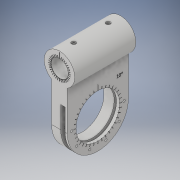
# Autodesk Inventor part: cam_holder_wrist_part
Saved by Autodesk Inventor 2019 (Build 230136000, 136)
## iProperties
Created: 2024-08-06
Part Number: cam_holder_wrist_part
Material: Generisch
Document SubType Name: Modeling
Designer: nic
Density: 1 g/cm^3
Appearance: Vorgabe
Author: nic
Autodesk Inventor part; units mm, degrees
ref_plane "YZ Plane" through (0, 0, 0) normal (1, 0, 0) x (0, 1, 0)
ref_plane "XY Plane" through (0, 0, 0) normal (0, 0, 1) x (1, 0, 0)
sketch "Skizze1" plane through (0, 0, 0) normal (1, 0, 0) x (0, 1, 0)
  line L0 (0, 0) -> (0, 35) construction
  circle A0 centre (0, 35) radius 35
  circle A1 centre (0, 35) radius 25.05
  dimension "d0" = 35
  dimension "d1" = 50.1
  constraints: 2 coincident, 2 end point, 1 centre point, 1 vertical, 1 vertical alignment, 2 other
  measures "d0" distance of L0.start L0.end
  measures "d1" diameter of A1
extrude "Extrusion1" add sketch "Skizze1" along normal blind 18
sketch "Skizze2" plane through (0, 0, 0) normal (0, 0, 1) x (1, 0, 0)
  line L0 (18, -35) -> (18, 35) construction
  line L1 (0, 35) -> (0, -35) construction
  line L2 (0, 35) -> (18, 35) projected
  line L3 (9, 35) -> (9, 60) construction
  circle A0 centre (9, 60) radius 10.05
  circle A1 centre (9, 60) radius 17.5
  point P0 (0, 0)
  dimension "d5" = 25
  dimension "d6" = 20.1
  dimension "d7" = 35
  constraints: 2 centre point, 2 coincident, 2 end point, 1 midpoint, 1 vertical
  measures "d5" distance of L3.start L3.end
  measures "d6" diameter of A0
  measures "d7" diameter of A1
extrude "Extrusion2" add sketch "Skizze2" along normal blind 70
sketch "Skizze3" plane through (0, 0, 0) normal (0, 0, 1) x (1, 0, 0)
  line L0 (18, -35) -> (18, 35) construction
  line L1 (0, 35) -> (0, -35) construction
  circle A0 centre (9, 60) radius 17.5 construction
  line L2 (18, -35) -> (18, 35) projected
  line L3 (18, 0) -> (0, 0)
  line L4 (0, 0) -> (0, 44.9917)
  line L5 (18, 44.9917) -> (18, 0)
  arc A1 (0, 44.9917) -> (18, 44.9917) centre (9, 60) ccw
  point P0 (0, 0)
  constraints: 6 end point, 2 point on circle, 1 centre point, 1 coincident, 1 horizontal, 1 midpoint, 1 parallel, 1 perpendicular, 2 other
extrude "Extrusion3" add sketch "Skizze3" along normal blind 70
sketch "Skizze4" plane through (0, 0, 0) normal (-1, 0, 0) x (0, 0, 1)
  line L0 (9.95, 0) -> (60.05, 0) projected
  circle A0 centre (35, 0) radius 25.05
  point P0 (0, 0)
  constraints: 1 centre point, 1 midpoint
extrude "Extrusion4" cut sketch "Skizze4" against normal through all
ref_plane "Arbeitsebene1" through (13, 0, 0) normal (1, 0, 0) x (0, 0, -1)
sketch "Skizze5" plane through (13, 0, 0) normal (1, 0, 0) x (0, 0, -1)
  circle A0 centre (-35, 0) radius 25.05 construction
  arc A1 (-70, 0) -> (0, 0) centre (-35, 0) ccw construction
  line L0 (0, 44.9917) -> (0, 0) construction
  line L1 (-70, 44.9917) -> (0, 44.9917) construction
  line L2 (-70, 0) -> (-70, 44.9917) construction
  circle A2 centre (-35, 0) radius 25.05
  arc A3 (-59.4438, 25.05) -> (-10.5562, 25.05) centre (-35, 0) ccw
  line L3 (-70, 0) -> (-70, 44.9917) projected
  line L4 (-70, 25.05) -> (0, 25.05)
  line L5 (0, 25.05) -> (0, 0)
  line L6 (-70, 0) -> (-70, 25.05)
  constraints: 6 end point, 4 point on circle, 3 point on line, 2 centre point, 2 coincident, 1 horizontal, 1 parallel, 1 perpendicular
extrude "Extrusion5" cut sketch "Skizze5" against normal blind 1.325 and the other way blind 1.325
sketch "Skizze6" plane through (13, 0, 0) normal (1, 0, 0) x (0, 0, -1)
  circle A0 centre (-35, 0) radius 25.05 construction
  arc A1 (-70, 0) -> (0, 0) centre (-35, 0) ccw construction
  line L0 (0, 44.9917) -> (0, 0) construction
  line L1 (-70, 44.9917) -> (0, 44.9917) construction
  line L2 (-70, 0) -> (-70, 44.9917) construction
  arc A2 (-70, 0) -> (0, 0) centre (-35, 0) ccw projected
  line L3 (-70, 25.05) -> (-70, 0) projected
  line L4 (0, 0) -> (0, 25.05) projected
  line L5 (-70, 25.05) -> (-35, 25.05) projected
  line L6 (-35, 25.05) -> (0, 25.05) projected
  line L7 (-65, 39.9917) -> (-5, 39.9917)
  line L8 (-5, 39.9917) -> (-5, 0)
  arc A3 (-65, 0) -> (-5, 0) centre (-35, 0) ccw
  line L9 (-65, 0) -> (-65, 39.9917)
  line L10 (-65, 25.05) -> (-5, 25.05)
  dimension "d19" = 5
  constraints: 8 end point, 4 point on line, 2 point on circle, 1 centre point, 1 vertical alignment, 3 other
  measures "d19" distance between parallel lines of L2 L9
extrude "Extrusion6" cut sketch "Skizze6" against normal blind 2.5 and the other way blind 2.5 contours L3 L5 L9 A3 L8 L6 L4 A2
ref_plane "Arbeitsebene2" through (0, 78, 0) normal (0, 1, 0) x (-1, 0, 0)
sketch "Skizze7" plane through (0, 78, 0) normal (0, 1, 0) x (-1, 0, 0)
  line L0 (-19.05, 70) -> (1.05, 70) projected
  line L1 (-9, 70) -> (-9, 0)
  point P0 (0, 0)
  point P1 (-9, 53.6501)
  point P2 (-9, 14.2598)
  constraints: 2 end point, 2 point on line, 1 midpoint, 1 vertical
hole "Bohrung1" at (9, 78, 53.6501) at (9, 78, 14.2598) direction (0, -1, 0) diameter 3.8 depth 10 tip angle 118 counterbore diameter 5 counterbore depth 2
sketch "Skizze8" plane through (0, 0, 70) normal (0, 0, 1) x (1, 0, 0)
  circle A0 centre (9, 60) radius 10.05 construction
  arc A1 (18, 44.9917) -> (0, 44.9917) centre (9, 60) ccw construction
  line L0 (8.75, 67.55) -> (9.25, 67.55)
  line L1 (9.25, 67.55) -> (9.25, 72.55)
  line L2 (9.25, 72.55) -> (8.75, 72.55)
  line L3 (8.75, 72.55) -> (8.75, 67.55)
  line L4 (8.75, 67.55) -> (9.25, 72.55) construction
  line L5 (9.25, 67.55) -> (8.75, 72.55) construction
  line L6 (7.4428, 67.3919) -> (7.9352, 67.4787)
  line L7 (7.9352, 67.4787) -> (7.0669, 72.4027)
  line L8 (7.0669, 72.4027) -> (6.5745, 72.3159)
  line L9 (6.5745, 72.3159) -> (7.4428, 67.3919)
  line L10 (7.4428, 67.3919) -> (7.0669, 72.4027) construction
  line L11 (7.9352, 67.4787) -> (6.5745, 72.3159) construction
  line L12 (6.1828, 67.0092) -> (6.6527, 67.1802)
  line L13 (6.6527, 67.1802) -> (4.9426, 71.8786)
  line L14 (4.9426, 71.8786) -> (4.4727, 71.7076)
  line L15 (4.4727, 71.7076) -> (6.1828, 67.0092)
  line L16 (6.1828, 67.0092) -> (4.9426, 71.8786) construction
  line L17 (6.6527, 67.1802) -> (4.4727, 71.7076) construction
  line L18 (5.0085, 66.4135) -> (5.4415, 66.6635)
  line L19 (5.4415, 66.6635) -> (2.9415, 70.9936)
  line L20 (2.9415, 70.9936) -> (2.5085, 70.7436)
  line L21 (2.5085, 70.7436) -> (5.0085, 66.4135)
  line L22 (5.0085, 66.4135) -> (2.9415, 70.9936) construction
  line L23 (5.4415, 66.6635) -> (2.5085, 70.7436) construction
  line L24 (3.9554, 65.6229) -> (4.3385, 65.9443)
  line L25 (4.3385, 65.9443) -> (1.1245, 69.7746)
  line L26 (1.1245, 69.7746) -> (0.7415, 69.4532)
  line L27 (0.7415, 69.4532) -> (3.9554, 65.6229)
  line L28 (3.9554, 65.6229) -> (1.1245, 69.7746) construction
  line L29 (4.3385, 65.9443) -> (0.7415, 69.4532) construction
  line L30 (3.0557, 64.6615) -> (3.3771, 65.0446)
  line L31 (3.3771, 65.0446) -> (-0.4532, 68.2585)
  line L32 (-0.4532, 68.2585) -> (-0.7746, 67.8755)
  line L33 (-0.7746, 67.8755) -> (3.0557, 64.6615)
  line L34 (3.0557, 64.6615) -> (-0.4532, 68.2585) construction
  line L35 (3.3771, 65.0446) -> (-0.7746, 67.8755) construction
  line L36 (2.3365, 63.5585) -> (2.5865, 63.9915)
  line L37 (2.5865, 63.9915) -> (-1.7436, 66.4915)
  line L38 (-1.7436, 66.4915) -> (-1.9936, 66.0585)
  line L39 (-1.9936, 66.0585) -> (2.3365, 63.5585)
  line L40 (2.3365, 63.5585) -> (-1.7436, 66.4915) construction
  line L41 (2.5865, 63.9915) -> (-1.9936, 66.0585) construction
  line L42 (1.8198, 62.3473) -> (1.9908, 62.8172)
  line L43 (1.9908, 62.8172) -> (-2.7076, 64.5273)
  line L44 (-2.7076, 64.5273) -> (-2.8786, 64.0574)
  line L45 (-2.8786, 64.0574) -> (1.8198, 62.3473)
  line L46 (1.8198, 62.3473) -> (-2.7076, 64.5273) construction
  line L47 (1.9908, 62.8172) -> (-2.8786, 64.0574) construction
  line L48 (1.5213, 61.0648) -> (1.6081, 61.5572)
  line L49 (1.6081, 61.5572) -> (-3.3159, 62.4255)
  line L50 (-3.3159, 62.4255) -> (-3.4027, 61.9331)
  line L51 (-3.4027, 61.9331) -> (1.5213, 61.0648)
  line L52 (1.5213, 61.0648) -> (-3.3159, 62.4255) construction
  line L53 (1.6081, 61.5572) -> (-3.4027, 61.9331) construction
  line L54 (1.45, 59.75) -> (1.45, 60.25)
  line L55 (1.45, 60.25) -> (-3.55, 60.25)
  line L56 (-3.55, 60.25) -> (-3.55, 59.75)
  line L57 (-3.55, 59.75) -> (1.45, 59.75)
  line L58 (1.45, 59.75) -> (-3.55, 60.25) construction
  line L59 (1.45, 60.25) -> (-3.55, 59.75) construction
  line L60 (1.6081, 58.4428) -> (1.5213, 58.9352)
  line L61 (1.5213, 58.9352) -> (-3.4027, 58.0669)
  line L62 (-3.4027, 58.0669) -> (-3.3159, 57.5745)
  line L63 (-3.3159, 57.5745) -> (1.6081, 58.4428)
  line L64 (1.6081, 58.4428) -> (-3.4027, 58.0669) construction
  line L65 (1.5213, 58.9352) -> (-3.3159, 57.5745) construction
  line L66 (1.9908, 57.1828) -> (1.8198, 57.6527)
  line L67 (1.8198, 57.6527) -> (-2.8786, 55.9426)
  line L68 (-2.8786, 55.9426) -> (-2.7076, 55.4727)
  line L69 (-2.7076, 55.4727) -> (1.9908, 57.1828)
  line L70 (1.9908, 57.1828) -> (-2.8786, 55.9426) construction
  line L71 (1.8198, 57.6527) -> (-2.7076, 55.4727) construction
  line L72 (2.5865, 56.0085) -> (2.3365, 56.4415)
  line L73 (2.3365, 56.4415) -> (-1.9936, 53.9415)
  line L74 (-1.9936, 53.9415) -> (-1.7436, 53.5085)
  line L75 (-1.7436, 53.5085) -> (2.5865, 56.0085)
  line L76 (2.5865, 56.0085) -> (-1.9936, 53.9415) construction
  line L77 (2.3365, 56.4415) -> (-1.7436, 53.5085) construction
  line L78 (3.3771, 54.9554) -> (3.0557, 55.3385)
  line L79 (3.0557, 55.3385) -> (-0.7746, 52.1245)
  line L80 (-0.7746, 52.1245) -> (-0.4532, 51.7415)
  line L81 (-0.4532, 51.7415) -> (3.3771, 54.9554)
  line L82 (3.3771, 54.9554) -> (-0.7746, 52.1245) construction
  line L83 (3.0557, 55.3385) -> (-0.4532, 51.7415) construction
  line L84 (4.3385, 54.0557) -> (3.9554, 54.3771)
  line L85 (3.9554, 54.3771) -> (0.7415, 50.5468)
  line L86 (0.7415, 50.5468) -> (1.1245, 50.2254)
  line L87 (1.1245, 50.2254) -> (4.3385, 54.0557)
  line L88 (4.3385, 54.0557) -> (0.7415, 50.5468) construction
  line L89 (3.9554, 54.3771) -> (1.1245, 50.2254) construction
  line L90 (5.4415, 53.3365) -> (5.0085, 53.5865)
  line L91 (5.0085, 53.5865) -> (2.5085, 49.2564)
  line L92 (2.5085, 49.2564) -> (2.9415, 49.0064)
  line L93 (2.9415, 49.0064) -> (5.4415, 53.3365)
  line L94 (5.4415, 53.3365) -> (2.5085, 49.2564) construction
  line L95 (5.0085, 53.5865) -> (2.9415, 49.0064) construction
  line L96 (6.6527, 52.8198) -> (6.1828, 52.9908)
  line L97 (6.1828, 52.9908) -> (4.4727, 48.2924)
  line L98 (4.4727, 48.2924) -> (4.9426, 48.1214)
  line L99 (4.9426, 48.1214) -> (6.6527, 52.8198)
  line L100 (6.6527, 52.8198) -> (4.4727, 48.2924) construction
  line L101 (6.1828, 52.9908) -> (4.9426, 48.1214) construction
  line L102 (7.9352, 52.5213) -> (7.4428, 52.6081)
  line L103 (7.4428, 52.6081) -> (6.5745, 47.6841)
  line L104 (6.5745, 47.6841) -> (7.0669, 47.5973)
  line L105 (7.0669, 47.5973) -> (7.9352, 52.5213)
  line L106 (7.9352, 52.5213) -> (6.5745, 47.6841) construction
  line L107 (7.4428, 52.6081) -> (7.0669, 47.5973) construction
  line L108 (9.25, 52.45) -> (8.75, 52.45)
  line L109 (8.75, 52.45) -> (8.75, 47.45)
  line L110 (8.75, 47.45) -> (9.25, 47.45)
  line L111 (9.25, 47.45) -> (9.25, 52.45)
  line L112 (9.25, 52.45) -> (8.75, 47.45) construction
  line L113 (8.75, 52.45) -> (9.25, 47.45) construction
  line L114 (10.5572, 52.6081) -> (10.0648, 52.5213)
  line L115 (10.0648, 52.5213) -> (10.9331, 47.5973)
  line L116 (10.9331, 47.5973) -> (11.4255, 47.6841)
  line L117 (11.4255, 47.6841) -> (10.5572, 52.6081)
  line L118 (10.5572, 52.6081) -> (10.9331, 47.5973) construction
  line L119 (10.0648, 52.5213) -> (11.4255, 47.6841) construction
  line L120 (11.8172, 52.9908) -> (11.3473, 52.8198)
  line L121 (11.3473, 52.8198) -> (13.0574, 48.1214)
  line L122 (13.0574, 48.1214) -> (13.5273, 48.2924)
  line L123 (13.5273, 48.2924) -> (11.8172, 52.9908)
  line L124 (11.8172, 52.9908) -> (13.0574, 48.1214) construction
  line L125 (11.3473, 52.8198) -> (13.5273, 48.2924) construction
  line L126 (12.9915, 53.5865) -> (12.5585, 53.3365)
  line L127 (12.5585, 53.3365) -> (15.0585, 49.0064)
  line L128 (15.0585, 49.0064) -> (15.4915, 49.2564)
  line L129 (15.4915, 49.2564) -> (12.9915, 53.5865)
  line L130 (12.9915, 53.5865) -> (15.0585, 49.0064) construction
  line L131 (12.5585, 53.3365) -> (15.4915, 49.2564) construction
  line L132 (14.0446, 54.3771) -> (13.6615, 54.0557)
  line L133 (13.6615, 54.0557) -> (16.8755, 50.2254)
  line L134 (16.8755, 50.2254) -> (17.2585, 50.5468)
  line L135 (17.2585, 50.5468) -> (14.0446, 54.3771)
  line L136 (14.0446, 54.3771) -> (16.8755, 50.2254) construction
  line L137 (13.6615, 54.0557) -> (17.2585, 50.5468) construction
  line L138 (14.9443, 55.3385) -> (14.6229, 54.9554)
  line L139 (14.6229, 54.9554) -> (18.4532, 51.7415)
  line L140 (18.4532, 51.7415) -> (18.7746, 52.1245)
  line L141 (18.7746, 52.1245) -> (14.9443, 55.3385)
  line L142 (14.9443, 55.3385) -> (18.4532, 51.7415) construction
  line L143 (14.6229, 54.9554) -> (18.7746, 52.1245) construction
  line L144 (15.6635, 56.4415) -> (15.4135, 56.0085)
  line L145 (15.4135, 56.0085) -> (19.7436, 53.5085)
  line L146 (19.7436, 53.5085) -> (19.9936, 53.9415)
  line L147 (19.9936, 53.9415) -> (15.6635, 56.4415)
  line L148 (15.6635, 56.4415) -> (19.7436, 53.5085) construction
  line L149 (15.4135, 56.0085) -> (19.9936, 53.9415) construction
  line L150 (16.1802, 57.6527) -> (16.0092, 57.1828)
  line L151 (16.0092, 57.1828) -> (20.7076, 55.4727)
  line L152 (20.7076, 55.4727) -> (20.8786, 55.9426)
  line L153 (20.8786, 55.9426) -> (16.1802, 57.6527)
  line L154 (16.1802, 57.6527) -> (20.7076, 55.4727) construction
  line L155 (16.0092, 57.1828) -> (20.8786, 55.9426) construction
  line L156 (16.4787, 58.9352) -> (16.3919, 58.4428)
  line L157 (16.3919, 58.4428) -> (21.3159, 57.5745)
  line L158 (21.3159, 57.5745) -> (21.4027, 58.0669)
  line L159 (21.4027, 58.0669) -> (16.4787, 58.9352)
  line L160 (16.4787, 58.9352) -> (21.3159, 57.5745) construction
  line L161 (16.3919, 58.4428) -> (21.4027, 58.0669) construction
  line L162 (16.55, 60.25) -> (16.55, 59.75)
  line L163 (16.55, 59.75) -> (21.55, 59.75)
  line L164 (21.55, 59.75) -> (21.55, 60.25)
  line L165 (21.55, 60.25) -> (16.55, 60.25)
  line L166 (16.55, 60.25) -> (21.55, 59.75) construction
  line L167 (16.55, 59.75) -> (21.55, 60.25) construction
  line L168 (16.3919, 61.5572) -> (16.4787, 61.0648)
  line L169 (16.4787, 61.0648) -> (21.4027, 61.9331)
  line L170 (21.4027, 61.9331) -> (21.3159, 62.4255)
  line L171 (21.3159, 62.4255) -> (16.3919, 61.5572)
  line L172 (16.3919, 61.5572) -> (21.4027, 61.9331) construction
  line L173 (16.4787, 61.0648) -> (21.3159, 62.4255) construction
  line L174 (16.0092, 62.8172) -> (16.1802, 62.3473)
  line L175 (16.1802, 62.3473) -> (20.8786, 64.0574)
  line L176 (20.8786, 64.0574) -> (20.7076, 64.5273)
  line L177 (20.7076, 64.5273) -> (16.0092, 62.8172)
  line L178 (16.0092, 62.8172) -> (20.8786, 64.0574) construction
  line L179 (16.1802, 62.3473) -> (20.7076, 64.5273) construction
  line L180 (15.4135, 63.9915) -> (15.6635, 63.5585)
  line L181 (15.6635, 63.5585) -> (19.9936, 66.0585)
  line L182 (19.9936, 66.0585) -> (19.7436, 66.4915)
  line L183 (19.7436, 66.4915) -> (15.4135, 63.9915)
  line L184 (15.4135, 63.9915) -> (19.9936, 66.0585) construction
  line L185 (15.6635, 63.5585) -> (19.7436, 66.4915) construction
  line L186 (14.6229, 65.0446) -> (14.9443, 64.6615)
  line L187 (14.9443, 64.6615) -> (18.7746, 67.8755)
  line L188 (18.7746, 67.8755) -> (18.4532, 68.2585)
  line L189 (18.4532, 68.2585) -> (14.6229, 65.0446)
  line L190 (14.6229, 65.0446) -> (18.7746, 67.8755) construction
  line L191 (14.9443, 64.6615) -> (18.4532, 68.2585) construction
  line L192 (13.6615, 65.9443) -> (14.0446, 65.6229)
  line L193 (14.0446, 65.6229) -> (17.2585, 69.4532)
  line L194 (17.2585, 69.4532) -> (16.8755, 69.7746)
  line L195 (16.8755, 69.7746) -> (13.6615, 65.9443)
  line L196 (13.6615, 65.9443) -> (17.2585, 69.4532) construction
  line L197 (14.0446, 65.6229) -> (16.8755, 69.7746) construction
  line L198 (12.5585, 66.6635) -> (12.9915, 66.4135)
  line L199 (12.9915, 66.4135) -> (15.4915, 70.7436)
  line L200 (15.4915, 70.7436) -> (15.0585, 70.9936)
  line L201 (15.0585, 70.9936) -> (12.5585, 66.6635)
  line L202 (12.5585, 66.6635) -> (15.4915, 70.7436) construction
  line L203 (12.9915, 66.4135) -> (15.0585, 70.9936) construction
  line L204 (11.3473, 67.1802) -> (11.8172, 67.0092)
  line L205 (11.8172, 67.0092) -> (13.5273, 71.7076)
  line L206 (13.5273, 71.7076) -> (13.0574, 71.8786)
  line L207 (13.0574, 71.8786) -> (11.3473, 67.1802)
  line L208 (11.3473, 67.1802) -> (13.5273, 71.7076) construction
  line L209 (11.8172, 67.0092) -> (13.0574, 71.8786) construction
  line L210 (10.0648, 67.4787) -> (10.5572, 67.3919)
  line L211 (10.5572, 67.3919) -> (11.4255, 72.3159)
  line L212 (11.4255, 72.3159) -> (10.9331, 72.4027)
  line L213 (10.9331, 72.4027) -> (10.0648, 67.4787)
  line L214 (10.0648, 67.4787) -> (11.4255, 72.3159) construction
  line L215 (10.5572, 67.3919) -> (10.9331, 72.4027) construction
  point P0 (0, 0)
  point P1 (9, 70.05)
  point P2 (7.2548, 69.8973)
  point P3 (5.5627, 69.4439)
  point P4 (3.975, 68.7036)
  point P5 (2.54, 67.6987)
  point P6 (1.3013, 66.46)
  point P7 (0.2964, 65.025)
  point P8 (-0.4439, 63.4373)
  point P9 (-0.8973, 61.7452)
  point P10 (-1.05, 60)
  point P11 (-0.8973, 58.2548)
  point P12 (-0.4439, 56.5627)
  point P13 (0.2964, 54.975)
  point P14 (1.3013, 53.54)
  point P15 (2.54, 52.3013)
  point P16 (3.975, 51.2964)
  point P17 (5.5627, 50.5561)
  point P18 (7.2548, 50.1027)
  point P19 (9, 49.95)
  point P20 (10.7452, 50.1027)
  point P21 (12.4373, 50.5561)
  point P22 (14.025, 51.2964)
  point P23 (15.46, 52.3013)
  point P24 (16.6987, 53.54)
  point P25 (17.7036, 54.975)
  point P26 (18.4439, 56.5627)
  point P27 (18.8973, 58.2548)
  point P28 (19.05, 60)
  point P29 (18.8973, 61.7452)
  point P30 (18.4439, 63.4373)
  point P31 (17.7036, 65.025)
  point P32 (16.6987, 66.46)
  point P33 (15.46, 67.6987)
  point P34 (14.025, 68.7036)
  point P35 (12.4373, 69.4439)
  point P36 (10.7452, 69.8973)
  dimension "d32" = 0.5
  dimension "d33" = 5
  dimension "d36" = 360
  constraints: 432 end point, 72 midpoint, 2 parallel, 1 horizontal, 1 perpendicular, 1 vertical alignment, 398 other
  measures "d32" distance of L2.end L1.end
  measures "d33" distance of L1.end L0.end
extrude "Extrusion7" cut sketch "Skizze8" against normal blind 0.5
sketch "Skizze9" plane through (0, 0, 70) normal (0, 0, 1) x (1, 0, 0)
  line L0 (9.25, 72.55) -> (9.25, 70.0469) projected
  line L1 (8.75, 70.0469) -> (8.75, 72.55) projected
  line L2 (8.75, 72.55) -> (9.25, 72.55) projected
  line L3 (11.5, 76) -> (6.5, 76) projected
  line L4 (8.75, 69.1) -> (9.25, 69.1)
  line L5 (9.25, 69.1) -> (9.25, 76)
  line L6 (9.25, 76) -> (8.75, 76)
  line L7 (8.75, 76) -> (8.75, 69.1)
  line L8 (8.75, 69.1) -> (9.25, 76) construction
  line L9 (9.25, 69.1) -> (8.75, 76) construction
  point P0 (0, 0)
  point P1 (9, 72.55)
  constraints: 12 end point, 3 midpoint, 2 parallel, 1 horizontal, 1 perpendicular, 1 point on line
extrude "Extrusion8" cut sketch "Skizze9" against normal blind 0.5
sketch "Skizze10" plane through (0, 0, 0) normal (0, 0, -1) x (-1, 0, 0)
  circle A0 centre (-9, 60) radius 10.05 projected
  circle A1 centre (-9, 60) radius 9.95
  point P0 (0, 0)
  dimension "d42" = 0.1
  constraints: 1 centre point
  measures "d42" radial gap between concentric circles of A0 A1
extrude "Extrusion9" add sketch "Skizze10" against normal up to surface (69.5 mm away)
sketch "Skizze11" plane through (18, 0, 0) normal (1, 0, 0) x (0, 0, -1)
  circle A0 centre (-35, 0) radius 25.05 projected
  line L0 (-35.25, 22.55) -> (-34.75, 22.55)
  line L1 (-34.75, 22.55) -> (-34.75, 27.55)
  line L2 (-34.75, 27.55) -> (-35.25, 27.55)
  line L3 (-35.25, 27.55) -> (-35.25, 22.55)
  line L4 (-65, 25.05) -> (-35, 25.05) projected
  line L5 (-35.25, 22.55) -> (-34.75, 27.55) construction
  line L6 (-34.75, 22.55) -> (-35.25, 27.55) construction
  line L7 (-39.162, 22.164) -> (-38.6696, 22.2508)
  line L8 (-38.6696, 22.2508) -> (-39.5378, 27.1749)
  line L9 (-39.5378, 27.1749) -> (-40.0302, 27.088)
  line L10 (-40.0302, 27.088) -> (-39.162, 22.164)
  line L11 (-39.162, 22.164) -> (-39.5378, 27.1749) construction
  line L12 (-38.6696, 22.2508) -> (-40.0302, 27.088) construction
  line L13 (-42.9475, 21.1046) -> (-42.4776, 21.2756)
  line L14 (-42.4776, 21.2756) -> (-44.1877, 25.974)
  line L15 (-44.1877, 25.974) -> (-44.6576, 25.803)
  line L16 (-44.6576, 25.803) -> (-42.9475, 21.1046)
  line L17 (-42.9475, 21.1046) -> (-44.1877, 25.974) construction
  line L18 (-42.4776, 21.2756) -> (-44.6576, 25.803) construction
  line L19 (-46.4915, 19.4039) -> (-46.0585, 19.6539)
  line L20 (-46.0585, 19.6539) -> (-48.5585, 23.984)
  line L21 (-48.5585, 23.984) -> (-48.9915, 23.734)
  line L22 (-48.9915, 23.734) -> (-46.4915, 19.4039)
  line L23 (-46.4915, 19.4039) -> (-48.5585, 23.984) construction
  line L24 (-46.0585, 19.6539) -> (-48.9915, 23.734) construction
  line L25 (-49.6864, 17.1136) -> (-49.3033, 17.435)
  line L26 (-49.3033, 17.435) -> (-52.5173, 21.2652)
  line L27 (-52.5173, 21.2652) -> (-52.9003, 20.9438)
  line L28 (-52.9003, 20.9438) -> (-49.6864, 17.1136)
  line L29 (-49.6864, 17.1136) -> (-52.5173, 21.2652) construction
  line L30 (-49.3033, 17.435) -> (-52.9003, 20.9438) construction
  line L31 (-52.435, 14.3033) -> (-52.1136, 14.6864)
  line L32 (-52.1136, 14.6864) -> (-55.9438, 17.9003)
  line L33 (-55.9438, 17.9003) -> (-56.2652, 17.5173)
  line L34 (-56.2652, 17.5173) -> (-52.435, 14.3033)
  line L35 (-52.435, 14.3033) -> (-55.9438, 17.9003) construction
  line L36 (-52.1136, 14.6864) -> (-56.2652, 17.5173) construction
  line L37 (-54.6539, 11.0585) -> (-54.4039, 11.4915)
  line L38 (-54.4039, 11.4915) -> (-58.734, 13.9915)
  line L39 (-58.734, 13.9915) -> (-58.984, 13.5585)
  line L40 (-58.984, 13.5585) -> (-54.6539, 11.0585)
  line L41 (-54.6539, 11.0585) -> (-58.734, 13.9915) construction
  line L42 (-54.4039, 11.4915) -> (-58.984, 13.5585) construction
  line L43 (-56.2756, 7.4776) -> (-56.1046, 7.9475)
  line L44 (-56.1046, 7.9475) -> (-60.803, 9.6576)
  line L45 (-60.803, 9.6576) -> (-60.974, 9.1877)
  line L46 (-60.974, 9.1877) -> (-56.2756, 7.4776)
  line L47 (-56.2756, 7.4776) -> (-60.803, 9.6576) construction
  line L48 (-56.1046, 7.9475) -> (-60.974, 9.1877) construction
  line L49 (-57.2508, 3.6696) -> (-57.164, 4.162)
  line L50 (-57.164, 4.162) -> (-62.088, 5.0302)
  line L51 (-62.088, 5.0302) -> (-62.1749, 4.5378)
  line L52 (-62.1749, 4.5378) -> (-57.2508, 3.6696)
  line L53 (-57.2508, 3.6696) -> (-62.088, 5.0302) construction
  line L54 (-57.164, 4.162) -> (-62.1749, 4.5378) construction
  line L55 (-57.55, -0.25) -> (-57.55, 0.25)
  line L56 (-57.55, 0.25) -> (-62.55, 0.25)
  line L57 (-62.55, 0.25) -> (-62.55, -0.25)
  line L58 (-62.55, -0.25) -> (-57.55, -0.25)
  line L59 (-57.55, -0.25) -> (-62.55, 0.25) construction
  line L60 (-57.55, 0.25) -> (-62.55, -0.25) construction
  line L61 (-57.164, -4.162) -> (-57.2508, -3.6696)
  line L62 (-57.2508, -3.6696) -> (-62.1749, -4.5378)
  line L63 (-62.1749, -4.5378) -> (-62.088, -5.0302)
  line L64 (-62.088, -5.0302) -> (-57.164, -4.162)
  line L65 (-57.164, -4.162) -> (-62.1749, -4.5378) construction
  line L66 (-57.2508, -3.6696) -> (-62.088, -5.0302) construction
  line L67 (-56.1046, -7.9475) -> (-56.2756, -7.4776)
  line L68 (-56.2756, -7.4776) -> (-60.974, -9.1877)
  line L69 (-60.974, -9.1877) -> (-60.803, -9.6576)
  line L70 (-60.803, -9.6576) -> (-56.1046, -7.9475)
  line L71 (-56.1046, -7.9475) -> (-60.974, -9.1877) construction
  line L72 (-56.2756, -7.4776) -> (-60.803, -9.6576) construction
  line L73 (-54.4039, -11.4915) -> (-54.6539, -11.0585)
  line L74 (-54.6539, -11.0585) -> (-58.984, -13.5585)
  line L75 (-58.984, -13.5585) -> (-58.734, -13.9915)
  line L76 (-58.734, -13.9915) -> (-54.4039, -11.4915)
  line L77 (-54.4039, -11.4915) -> (-58.984, -13.5585) construction
  line L78 (-54.6539, -11.0585) -> (-58.734, -13.9915) construction
  line L79 (-52.1136, -14.6864) -> (-52.435, -14.3033)
  line L80 (-52.435, -14.3033) -> (-56.2652, -17.5173)
  line L81 (-56.2652, -17.5173) -> (-55.9438, -17.9003)
  line L82 (-55.9438, -17.9003) -> (-52.1136, -14.6864)
  line L83 (-52.1136, -14.6864) -> (-56.2652, -17.5173) construction
  line L84 (-52.435, -14.3033) -> (-55.9438, -17.9003) construction
  line L85 (-49.3033, -17.435) -> (-49.6864, -17.1136)
  line L86 (-49.6864, -17.1136) -> (-52.9003, -20.9438)
  line L87 (-52.9003, -20.9438) -> (-52.5173, -21.2652)
  line L88 (-52.5173, -21.2652) -> (-49.3033, -17.435)
  line L89 (-49.3033, -17.435) -> (-52.9003, -20.9438) construction
  line L90 (-49.6864, -17.1136) -> (-52.5173, -21.2652) construction
  line L91 (-46.0585, -19.6539) -> (-46.4915, -19.4039)
  line L92 (-46.4915, -19.4039) -> (-48.9915, -23.734)
  line L93 (-48.9915, -23.734) -> (-48.5585, -23.984)
  line L94 (-48.5585, -23.984) -> (-46.0585, -19.6539)
  line L95 (-46.0585, -19.6539) -> (-48.9915, -23.734) construction
  line L96 (-46.4915, -19.4039) -> (-48.5585, -23.984) construction
  line L97 (-42.4776, -21.2756) -> (-42.9475, -21.1046)
  line L98 (-42.9475, -21.1046) -> (-44.6576, -25.803)
  line L99 (-44.6576, -25.803) -> (-44.1877, -25.974)
  line L100 (-44.1877, -25.974) -> (-42.4776, -21.2756)
  line L101 (-42.4776, -21.2756) -> (-44.6576, -25.803) construction
  line L102 (-42.9475, -21.1046) -> (-44.1877, -25.974) construction
  line L103 (-38.6696, -22.2508) -> (-39.162, -22.164)
  line L104 (-39.162, -22.164) -> (-40.0302, -27.088)
  line L105 (-40.0302, -27.088) -> (-39.5378, -27.1749)
  line L106 (-39.5378, -27.1749) -> (-38.6696, -22.2508)
  line L107 (-38.6696, -22.2508) -> (-40.0302, -27.088) construction
  line L108 (-39.162, -22.164) -> (-39.5378, -27.1749) construction
  line L109 (-34.75, -22.55) -> (-35.25, -22.55)
  line L110 (-35.25, -22.55) -> (-35.25, -27.55)
  line L111 (-35.25, -27.55) -> (-34.75, -27.55)
  line L112 (-34.75, -27.55) -> (-34.75, -22.55)
  line L113 (-34.75, -22.55) -> (-35.25, -27.55) construction
  line L114 (-35.25, -22.55) -> (-34.75, -27.55) construction
  line L115 (-30.838, -22.164) -> (-31.3304, -22.2508)
  line L116 (-31.3304, -22.2508) -> (-30.4622, -27.1749)
  line L117 (-30.4622, -27.1749) -> (-29.9698, -27.088)
  line L118 (-29.9698, -27.088) -> (-30.838, -22.164)
  line L119 (-30.838, -22.164) -> (-30.4622, -27.1749) construction
  line L120 (-31.3304, -22.2508) -> (-29.9698, -27.088) construction
  line L121 (-27.0525, -21.1046) -> (-27.5224, -21.2756)
  line L122 (-27.5224, -21.2756) -> (-25.8123, -25.974)
  line L123 (-25.8123, -25.974) -> (-25.3424, -25.803)
  line L124 (-25.3424, -25.803) -> (-27.0525, -21.1046)
  line L125 (-27.0525, -21.1046) -> (-25.8123, -25.974) construction
  line L126 (-27.5224, -21.2756) -> (-25.3424, -25.803) construction
  line L127 (-23.5085, -19.4039) -> (-23.9415, -19.6539)
  line L128 (-23.9415, -19.6539) -> (-21.4415, -23.984)
  line L129 (-21.4415, -23.984) -> (-21.0085, -23.734)
  line L130 (-21.0085, -23.734) -> (-23.5085, -19.4039)
  line L131 (-23.5085, -19.4039) -> (-21.4415, -23.984) construction
  line L132 (-23.9415, -19.6539) -> (-21.0085, -23.734) construction
  line L133 (-20.3136, -17.1136) -> (-20.6967, -17.435)
  line L134 (-20.6967, -17.435) -> (-17.4827, -21.2652)
  line L135 (-17.4827, -21.2652) -> (-17.0997, -20.9438)
  line L136 (-17.0997, -20.9438) -> (-20.3136, -17.1136)
  line L137 (-20.3136, -17.1136) -> (-17.4827, -21.2652) construction
  line L138 (-20.6967, -17.435) -> (-17.0997, -20.9438) construction
  line L139 (-17.565, -14.3033) -> (-17.8864, -14.6864)
  line L140 (-17.8864, -14.6864) -> (-14.0562, -17.9003)
  line L141 (-14.0562, -17.9003) -> (-13.7348, -17.5173)
  line L142 (-13.7348, -17.5173) -> (-17.565, -14.3033)
  line L143 (-17.565, -14.3033) -> (-14.0562, -17.9003) construction
  line L144 (-17.8864, -14.6864) -> (-13.7348, -17.5173) construction
  line L145 (-15.3461, -11.0585) -> (-15.5961, -11.4915)
  line L146 (-15.5961, -11.4915) -> (-11.266, -13.9915)
  line L147 (-11.266, -13.9915) -> (-11.016, -13.5585)
  line L148 (-11.016, -13.5585) -> (-15.3461, -11.0585)
  line L149 (-15.3461, -11.0585) -> (-11.266, -13.9915) construction
  line L150 (-15.5961, -11.4915) -> (-11.016, -13.5585) construction
  line L151 (-13.7244, -7.4776) -> (-13.8954, -7.9475)
  line L152 (-13.8954, -7.9475) -> (-9.197, -9.6576)
  line L153 (-9.197, -9.6576) -> (-9.026, -9.1877)
  line L154 (-9.026, -9.1877) -> (-13.7244, -7.4776)
  line L155 (-13.7244, -7.4776) -> (-9.197, -9.6576) construction
  line L156 (-13.8954, -7.9475) -> (-9.026, -9.1877) construction
  line L157 (-12.7492, -3.6696) -> (-12.836, -4.162)
  line L158 (-12.836, -4.162) -> (-7.912, -5.0302)
  line L159 (-7.912, -5.0302) -> (-7.8251, -4.5378)
  line L160 (-7.8251, -4.5378) -> (-12.7492, -3.6696)
  line L161 (-12.7492, -3.6696) -> (-7.912, -5.0302) construction
  line L162 (-12.836, -4.162) -> (-7.8251, -4.5378) construction
  line L163 (-12.45, 0.25) -> (-12.45, -0.25)
  line L164 (-12.45, -0.25) -> (-7.45, -0.25)
  line L165 (-7.45, -0.25) -> (-7.45, 0.25)
  line L166 (-7.45, 0.25) -> (-12.45, 0.25)
  line L167 (-12.45, 0.25) -> (-7.45, -0.25) construction
  line L168 (-12.45, -0.25) -> (-7.45, 0.25) construction
  line L169 (-12.836, 4.162) -> (-12.7492, 3.6696)
  line L170 (-12.7492, 3.6696) -> (-7.8251, 4.5378)
  line L171 (-7.8251, 4.5378) -> (-7.912, 5.0302)
  line L172 (-7.912, 5.0302) -> (-12.836, 4.162)
  line L173 (-12.836, 4.162) -> (-7.8251, 4.5378) construction
  line L174 (-12.7492, 3.6696) -> (-7.912, 5.0302) construction
  line L175 (-13.8954, 7.9475) -> (-13.7244, 7.4776)
  line L176 (-13.7244, 7.4776) -> (-9.026, 9.1877)
  line L177 (-9.026, 9.1877) -> (-9.197, 9.6576)
  line L178 (-9.197, 9.6576) -> (-13.8954, 7.9475)
  line L179 (-13.8954, 7.9475) -> (-9.026, 9.1877) construction
  line L180 (-13.7244, 7.4776) -> (-9.197, 9.6576) construction
  line L181 (-15.5961, 11.4915) -> (-15.3461, 11.0585)
  line L182 (-15.3461, 11.0585) -> (-11.016, 13.5585)
  line L183 (-11.016, 13.5585) -> (-11.266, 13.9915)
  line L184 (-11.266, 13.9915) -> (-15.5961, 11.4915)
  line L185 (-15.5961, 11.4915) -> (-11.016, 13.5585) construction
  line L186 (-15.3461, 11.0585) -> (-11.266, 13.9915) construction
  line L187 (-17.8864, 14.6864) -> (-17.565, 14.3033)
  line L188 (-17.565, 14.3033) -> (-13.7348, 17.5173)
  line L189 (-13.7348, 17.5173) -> (-14.0562, 17.9003)
  line L190 (-14.0562, 17.9003) -> (-17.8864, 14.6864)
  line L191 (-17.8864, 14.6864) -> (-13.7348, 17.5173) construction
  line L192 (-17.565, 14.3033) -> (-14.0562, 17.9003) construction
  line L193 (-20.6967, 17.435) -> (-20.3136, 17.1136)
  line L194 (-20.3136, 17.1136) -> (-17.0997, 20.9438)
  line L195 (-17.0997, 20.9438) -> (-17.4827, 21.2652)
  line L196 (-17.4827, 21.2652) -> (-20.6967, 17.435)
  line L197 (-20.6967, 17.435) -> (-17.0997, 20.9438) construction
  line L198 (-20.3136, 17.1136) -> (-17.4827, 21.2652) construction
  line L199 (-23.9415, 19.6539) -> (-23.5085, 19.4039)
  line L200 (-23.5085, 19.4039) -> (-21.0085, 23.734)
  line L201 (-21.0085, 23.734) -> (-21.4415, 23.984)
  line L202 (-21.4415, 23.984) -> (-23.9415, 19.6539)
  line L203 (-23.9415, 19.6539) -> (-21.0085, 23.734) construction
  line L204 (-23.5085, 19.4039) -> (-21.4415, 23.984) construction
  line L205 (-27.5224, 21.2756) -> (-27.0525, 21.1046)
  line L206 (-27.0525, 21.1046) -> (-25.3424, 25.803)
  line L207 (-25.3424, 25.803) -> (-25.8123, 25.974)
  line L208 (-25.8123, 25.974) -> (-27.5224, 21.2756)
  line L209 (-27.5224, 21.2756) -> (-25.3424, 25.803) construction
  line L210 (-27.0525, 21.1046) -> (-25.8123, 25.974) construction
  line L211 (-31.3304, 22.2508) -> (-30.838, 22.164)
  line L212 (-30.838, 22.164) -> (-29.9698, 27.088)
  line L213 (-29.9698, 27.088) -> (-30.4622, 27.1749)
  line L214 (-30.4622, 27.1749) -> (-31.3304, 22.2508)
  line L215 (-31.3304, 22.2508) -> (-29.9698, 27.088) construction
  line L216 (-30.838, 22.164) -> (-30.4622, 27.1749) construction
  line L217 (-34.75, 19.2227) -> (-35.25, 19.2227)
  line L218 (-35.25, 19.2227) -> (-35.25, 30.8773)
  line L219 (-35.25, 30.8773) -> (-34.75, 30.8773)
  line L220 (-34.75, 30.8773) -> (-34.75, 19.2227)
  line L221 (-34.75, 19.2227) -> (-35.25, 30.8773) construction
  line L222 (-35.25, 19.2227) -> (-34.75, 30.8773) construction
  point P0 (0, 0)
  dimension "d45" = 0.5
  dimension "d46" = 5
  dimension "d49" = 360
  constraints: 444 end point, 4 midpoint, 4 parallel, 2 horizontal, 2 perpendicular, 1 vertical alignment, 361 other
  measures "d45" distance of L2.end L1.end
  measures "d46" distance of L1.end L0.end
extrude "Extrusion10" cut sketch "Skizze11" against normal blind 0.5 contours A0 L164 L163 L166 | A0 L166 L165 L164 | L170 L169 L172 A0 | A0 L172 L171 L170 | L160 L159 L158 A0 | A0 L158 L157 L160 | L176 L175 L178 A0 | A0 L178 L177 L176 | L154 L153 L152 A0 | A0 L152 L151 L154 | L182 L181 L184 A0 | A0 L184 L183 L182 | L148 L147 L146 A0 | A0 L146 L145 L148 | L188 L187 L190 A0 | A0 L190 L189 L188 | L142 L141 L140 A0 | A0 L140 L139 L142 | L194 L193 L196 A0 | A0 L196 L195 L194 | L136 L135 L134 A0 | A0 L134 L133 L136 | L200 L199 L202 A0 | A0 L202 L201 L200 | L130 L129 L128 A0 | A0 L128 L127 L130 | L206 L205 L208 A0 | A0 L208 L207 L206 | L124 L123 L122 A0 | A0 L122 L121 L124 | L212 L211 L214 A0 | A0 L214 L213 L212 | L118 L117 L116 A0 | A0 L116 L115 L118 | L1 L0 L3 A0 | A0 L3 L2 L1 | L112 L111 L110 A0 | A0 L110 L109 L112 | L220 L217 L218 L0 | L2 L218 L219 L220 | L106 L105 L104 A0 | A0 L104 L103 L106 | L8 L7 L10 A0 | A0 L10 L4 L8 | L4 L10 L9 L8 | L100 L99 L98 A0 | A0 L98 L97 L100 | L14 L13 L16 A0 | A0 L16 L4 L14 | L4 L16 L15 L14 | L94 L93 L92 A0 | A0 L92 L91 L94 | L20 L19 L22 A0 | A0 L22 L21 L20 | L88 L87 L86 A0 | A0 L86 L85 L88 | L26 L25 L28 A0 | A0 L28 L27 L26 | L82 L81 L80 A0 | A0 L80 L79 L82 | L32 L31 L34 A0 | A0 L34 L33 L32 | L76 L75 L74 A0 | A0 L74 L73 L76 | L38 L37 L40 A0 | A0 L40 L39 L38 | L70 L69 L68 A0 | A0 L68 L67 L70 | L44 L43 L46 A0 | A0 L46 L45 L44 | L64 L63 L62 A0 | A0 L62 L61 L64 | L50 L49 L52 A0 | A0 L52 L51 L50 | L58 L57 L56 A0 | A0 L56 L55 L58
sketch "Skizze12" plane through (18, 0, 0) normal (1, 0, 0) x (0, 0, -1)
  line L0 (-13.6205, 29.8927) -> (-6.1014, 29.8927) construction
  line L1 (-6.1014, 29.8927) -> (-6.1014, 26.2481) construction
  line L2 (-6.1014, 26.2481) -> (-13.6205, 26.2481) construction
  line L3 (-13.6205, 26.2481) -> (-13.6205, 29.8927) construction
  line L4 (-11.3826, 26.3218) -> (-13.0901, 26.3218)
  line L5 (-13.0901, 26.3218) -> (-13.0901, 26.6792)
  line L6 (-13.0901, 26.6792) -> (-12.4548, 26.6792)
  line L7 (-12.4548, 26.6792) -> (-12.4548, 29.0248)
  line L8 (-12.4548, 29.0248) -> (-13.0901, 29.0248)
  line L9 (-13.0901, 29.0248) -> (-13.0901, 29.3453)
  spline S0 degree 2 poles (-13.0901, 29.3453) (-12.7299, 29.3453) (-12.3895, 29.5495) (-12.3668, 29.8332) knots 0 0 0 1 2 2 2
  line L10 (-12.3668, 29.8332) -> (-12.0038, 29.8332)
  line L11 (-12.0038, 29.8332) -> (-12.0038, 26.6792)
  line L12 (-12.0038, 26.6792) -> (-11.3826, 26.6792)
  line L13 (-11.3826, 26.6792) -> (-11.3826, 26.3218)
  spline S1 degree 2 poles (-8.5605, 28.0718) (-8.5605, 27.1302) (-9.1079, 26.2481) (-9.678, 26.2481) knots 0 0 0 1 2 2 2
  spline S2 degree 2 poles (-9.678, 26.2481) (-10.2566, 26.2481) (-10.7984, 27.1472) (-10.7984, 28.069) knots 0 0 0 1 2 2 2
  spline S3 degree 2 poles (-10.7984, 28.069) (-10.7984, 29.0163) (-10.2509, 29.8927) (-9.678, 29.8927) knots 0 0 0 1 2 2 2
  spline S4 degree 2 poles (-9.678, 29.8927) (-9.1022, 29.8927) (-8.5605, 28.9851) (-8.5605, 28.0718) knots 0 0 0 1 2 2 2
  spline S5 degree 2 poles (-9.1618, 27.0054) (-9.0937, 27.1784) (-9.037, 27.7116) (-9.037, 28.0718) knots 0 0 0 1 2 2 2
  spline S6 degree 2 poles (-9.037, 28.0718) (-9.037, 28.432) (-9.0937, 28.9624) (-9.1646, 29.1411) knots 0 0 0 1 2 2 2
  spline S7 degree 2 poles (-9.1646, 29.1411) (-9.2355, 29.3198) (-9.4823, 29.5041) (-9.678, 29.5041) knots 0 0 0 1 2 2 2
  spline S8 degree 2 poles (-9.678, 29.5041) (-9.8737, 29.5041) (-10.1261, 29.3198) (-10.1999, 29.1354) knots 0 0 0 1 2 2 2
  spline S9 degree 2 poles (-10.1999, 29.1354) (-10.2708, 28.9567) (-10.3219, 28.4122) (-10.3219, 28.069) knots 0 0 0 1 2 2 2
  spline S10 degree 2 poles (-10.3219, 28.069) (-10.3219, 27.7003) (-10.2765, 27.2067) (-10.2027, 27.0139) knots 0 0 0 1 2 2 2
  spline S11 degree 2 poles (-10.2027, 27.0139) (-10.1347, 26.8323) (-9.8822, 26.6366) (-9.678, 26.6366) knots 0 0 0 1 2 2 2
  spline S12 degree 2 poles (-9.678, 26.6366) (-9.4851, 26.6366) (-9.2327, 26.821) (-9.1618, 27.0054) knots 0 0 0 1 2 2 2
  spline S13 degree 2 poles (-6.3397, 28.9879) (-6.3397, 28.6107) (-6.8559, 28.0945) (-7.2331, 28.0945) knots 0 0 0 1 2 2 2
  spline S14 degree 2 poles (-7.2331, 28.0945) (-7.6075, 28.0945) (-8.1294, 28.6079) (-8.1294, 28.9879) knots 0 0 0 1 2 2 2
  spline S15 degree 2 poles (-8.1294, 28.9879) (-8.1294, 29.3652) (-7.6132, 29.8814) (-7.2331, 29.8814) knots 0 0 0 1 2 2 2
  spline S16 degree 2 poles (-7.2331, 29.8814) (-6.8559, 29.8814) (-6.3397, 29.3652) (-6.3397, 28.9879) knots 0 0 0 1 2 2 2
  spline S17 degree 2 poles (-6.7084, 28.9879) (-6.7084, 29.2148) (-7.009, 29.524) (-7.2331, 29.524) knots 0 0 0 1 2 2 2
  spline S18 degree 2 poles (-7.2331, 29.524) (-7.46, 29.524) (-7.7607, 29.2148) (-7.7607, 28.9879) knots 0 0 0 1 2 2 2
  spline S19 degree 2 poles (-7.7607, 28.9879) (-7.7607, 28.7582) (-7.4543, 28.4519) (-7.2331, 28.4519) knots 0 0 0 1 2 2 2
  spline S20 degree 2 poles (-7.2331, 28.4519) (-7.009, 28.4519) (-6.7084, 28.7639) (-6.7084, 28.9879) knots 0 0 0 1 2 2 2
  point P0 (0, 0)
  constraints: 2 other
extrude "Extrusion11" cut sketch "Skizze12" against normal blind 0.5
sketch "Skizze13" plane through (18, 0, 0) normal (1, 0, 0) x (0, 0, -1)
  line L0 (-11.3826, 26.6792) -> (-11.3826, 26.3218) construction
  line L1 (-11.3826, 26.3218) -> (-13.0901, 26.3218) construction
  line L2 (-13.0901, 26.3218) -> (-13.0901, 26.6792) construction
  line L3 (-13.0901, 26.6792) -> (-12.4548, 26.6792) construction
  line L4 (-12.4548, 26.6792) -> (-12.4548, 29.0248) construction
  line L5 (-12.4548, 29.0248) -> (-13.0901, 29.0248) construction
  line L6 (-13.0901, 29.0248) -> (-13.0901, 29.3453) construction
  line L7 (-12.3668, 29.8332) -> (-12.0038, 29.8332) construction
  line L8 (-12.0038, 29.8332) -> (-12.0038, 26.6792) construction
  line L9 (-12.0038, 26.6792) -> (-11.3826, 26.6792) construction
  line L10 (-29.9698, 27.088) -> (-30.4041, 24.6248) construction
  arc A0 (-26.6677, 23.6236) -> (-30.4041, 24.6248) centre (-35, 0) ccw construction
  line L11 (-26.6677, 23.6236) -> (-25.8123, 25.974) construction
  line L12 (-25.8123, 25.974) -> (-25.3424, 25.803) construction
  line L13 (-25.3424, 25.803) -> (-26.1979, 23.4526) construction
  arc A1 (-22.6921, 21.8179) -> (-26.1979, 23.4526) centre (-35, 0) ccw construction
  line L14 (-22.6921, 21.8179) -> (-21.4415, 23.984) construction
  line L15 (-21.4415, 23.984) -> (-21.0085, 23.734) construction
  line L16 (-21.0085, 23.734) -> (-22.2591, 21.5679) construction
  arc A2 (-19.0905, 19.3492) -> (-22.2591, 21.5679) centre (-35, 0) ccw construction
  line L17 (-19.0905, 19.3492) -> (-17.4827, 21.2652) construction
  line L18 (-17.4827, 21.2652) -> (-17.0997, 20.9438) construction
  line L19 (-17.0997, 20.9438) -> (-18.7075, 19.0278) construction
  arc A3 (-15.9722, 16.2925) -> (-18.7075, 19.0278) centre (-35, 0) ccw construction
  line L20 (-15.9722, 16.2925) -> (-14.0562, 17.9003) construction
  line L21 (-14.0562, 17.9003) -> (-13.7348, 17.5173) construction
  line L22 (-13.7348, 17.5173) -> (-15.6508, 15.9095) construction
  arc A4 (-13.4321, 12.7409) -> (-15.6508, 15.9095) centre (-35, 0) ccw construction
  line L23 (-13.4321, 12.7409) -> (-11.266, 13.9915) construction
  line L24 (-11.266, 13.9915) -> (-11.016, 13.5585) construction
  line L25 (-11.016, 13.5585) -> (-13.1821, 12.3079) construction
  arc A5 (-11.5474, 8.8021) -> (-13.1821, 12.3079) centre (-35, 0) ccw construction
  line L26 (-11.5474, 8.8021) -> (-9.197, 9.6576) construction
  line L27 (-9.197, 9.6576) -> (-9.026, 9.1877) construction
  line L28 (-9.026, 9.1877) -> (-11.3764, 8.3323) construction
  arc A6 (-10.3752, 4.5959) -> (-11.3764, 8.3323) centre (-35, 0) ccw construction
  line L29 (-10.3752, 4.5959) -> (-7.912, 5.0302) construction
  line L30 (-7.912, 5.0302) -> (-7.8251, 4.5378) construction
  line L31 (-7.8251, 4.5378) -> (-10.2884, 4.1035) construction
  arc A7 (-9.9512, 0.25) -> (-10.2884, 4.1035) centre (-35, 0) ccw construction
  line L32 (-9.9512, 0.25) -> (-7.45, 0.25) construction
  line L33 (-7.45, 0.25) -> (-7.45, -0.25) construction
  line L34 (-7.45, -0.25) -> (-9.9512, -0.25) construction
  arc A8 (-10.2884, -4.1035) -> (-9.9512, -0.25) centre (-35, 0) ccw construction
  line L35 (-10.2884, -4.1035) -> (-7.8251, -4.5378) construction
  line L36 (-7.8251, -4.5378) -> (-7.912, -5.0302) construction
  line L37 (-7.912, -5.0302) -> (-10.3752, -4.5959) construction
  arc A9 (-11.3764, -8.3323) -> (-10.3752, -4.5959) centre (-35, 0) ccw construction
  line L38 (-11.3764, -8.3323) -> (-9.026, -9.1877) construction
  line L39 (-9.026, -9.1877) -> (-9.197, -9.6576) construction
  line L40 (-9.197, -9.6576) -> (-11.5474, -8.8021) construction
  arc A10 (-13.1821, -12.3079) -> (-11.5474, -8.8021) centre (-35, 0) ccw construction
  line L41 (-13.1821, -12.3079) -> (-11.016, -13.5585) construction
  line L42 (-11.016, -13.5585) -> (-11.266, -13.9915) construction
  line L43 (-11.266, -13.9915) -> (-13.4321, -12.7409) construction
  arc A11 (-15.6508, -15.9095) -> (-13.4321, -12.7409) centre (-35, 0) ccw construction
  line L44 (-15.6508, -15.9095) -> (-13.7348, -17.5173) construction
  line L45 (-13.7348, -17.5173) -> (-14.0562, -17.9003) construction
  line L46 (-14.0562, -17.9003) -> (-15.9722, -16.2925) construction
  arc A12 (-18.7075, -19.0278) -> (-15.9722, -16.2925) centre (-35, 0) ccw construction
  line L47 (-18.7075, -19.0278) -> (-17.0997, -20.9438) construction
  line L48 (-17.0997, -20.9438) -> (-17.4827, -21.2652) construction
  line L49 (-17.4827, -21.2652) -> (-19.0905, -19.3492) construction
  arc A13 (-22.2591, -21.5679) -> (-19.0905, -19.3492) centre (-35, 0) ccw construction
  line L50 (-22.2591, -21.5679) -> (-21.0085, -23.734) construction
  line L51 (-21.0085, -23.734) -> (-21.4415, -23.984) construction
  line L52 (-21.4415, -23.984) -> (-22.6921, -21.8179) construction
  arc A14 (-26.1979, -23.4526) -> (-22.6921, -21.8179) centre (-35, 0) ccw construction
  line L53 (-26.1979, -23.4526) -> (-25.3424, -25.803) construction
  line L54 (-25.3424, -25.803) -> (-25.8123, -25.974) construction
  line L55 (-25.8123, -25.974) -> (-26.6677, -23.6236) construction
  arc A15 (-30.4041, -24.6248) -> (-26.6677, -23.6236) centre (-35, 0) ccw construction
  line L56 (-30.4041, -24.6248) -> (-29.9698, -27.088) construction
  line L57 (-29.9698, -27.088) -> (-30.4622, -27.1749) construction
  line L58 (-30.4622, -27.1749) -> (-30.8965, -24.7116) construction
  arc A16 (-34.75, -25.0488) -> (-30.8965, -24.7116) centre (-35, 0) ccw construction
  line L59 (-34.75, -25.0488) -> (-34.75, -27.55) construction
  line L60 (-34.75, -27.55) -> (-35.25, -27.55) construction
  line L61 (-35.25, -27.55) -> (-35.25, -25.0488) construction
  arc A17 (-39.1035, -24.7116) -> (-35.25, -25.0488) centre (-35, 0) ccw construction
  line L62 (-39.1035, -24.7116) -> (-39.5378, -27.1749) construction
  line L63 (-39.5378, -27.1749) -> (-40.0302, -27.088) construction
  line L64 (-40.0302, -27.088) -> (-39.5959, -24.6248) construction
  arc A18 (-43.3323, -23.6236) -> (-39.5959, -24.6248) centre (-35, 0) ccw construction
  line L65 (-43.3323, -23.6236) -> (-44.1877, -25.974) construction
  line L66 (-44.1877, -25.974) -> (-44.6576, -25.803) construction
  line L67 (-44.6576, -25.803) -> (-43.8021, -23.4526) construction
  arc A19 (-47.3079, -21.8179) -> (-43.8021, -23.4526) centre (-35, 0) ccw construction
  line L68 (-47.3079, -21.8179) -> (-48.5585, -23.984) construction
  line L69 (-48.5585, -23.984) -> (-48.9915, -23.734) construction
  line L70 (-48.9915, -23.734) -> (-47.7409, -21.5679) construction
  arc A20 (-50.9095, -19.3492) -> (-47.7409, -21.5679) centre (-35, 0) ccw construction
  line L71 (-50.9095, -19.3492) -> (-52.5173, -21.2652) construction
  line L72 (-52.5173, -21.2652) -> (-52.9003, -20.9438) construction
  line L73 (-52.9003, -20.9438) -> (-51.2925, -19.0278) construction
  arc A21 (-54.0278, -16.2925) -> (-51.2925, -19.0278) centre (-35, 0) ccw construction
  line L74 (-54.0278, -16.2925) -> (-55.9438, -17.9003) construction
  line L75 (-55.9438, -17.9003) -> (-56.2652, -17.5173) construction
  line L76 (-56.2652, -17.5173) -> (-54.3492, -15.9095) construction
  arc A22 (-56.5679, -12.7409) -> (-54.3492, -15.9095) centre (-35, 0) ccw construction
  line L77 (-56.5679, -12.7409) -> (-58.734, -13.9915) construction
  line L78 (-58.734, -13.9915) -> (-58.984, -13.5585) construction
  line L79 (-58.984, -13.5585) -> (-56.8179, -12.3079) construction
  arc A23 (-58.4526, -8.8021) -> (-56.8179, -12.3079) centre (-35, 0) ccw construction
  line L80 (-58.4526, -8.8021) -> (-60.803, -9.6576) construction
  line L81 (-60.803, -9.6576) -> (-60.974, -9.1877) construction
  line L82 (-60.974, -9.1877) -> (-58.6236, -8.3323) construction
  arc A24 (-59.6248, -4.5959) -> (-58.6236, -8.3323) centre (-35, 0) ccw construction
  line L83 (-59.6248, -4.5959) -> (-62.088, -5.0302) construction
  line L84 (-62.088, -5.0302) -> (-62.1749, -4.5378) construction
  line L85 (-62.1749, -4.5378) -> (-59.7116, -4.1035) construction
  arc A25 (-60.0488, -0.25) -> (-59.7116, -4.1035) centre (-35, 0) ccw construction
  line L86 (-60.0488, -0.25) -> (-62.55, -0.25) construction
  line L87 (-62.55, -0.25) -> (-62.55, 0.25) construction
  line L88 (-62.55, 0.25) -> (-60.0488, 0.25) construction
  arc A26 (-59.7116, 4.1035) -> (-60.0488, 0.25) centre (-35, 0) ccw construction
  line L89 (-59.7116, 4.1035) -> (-62.1749, 4.5378) construction
  line L90 (-62.1749, 4.5378) -> (-62.088, 5.0302) construction
  line L91 (-62.088, 5.0302) -> (-59.6248, 4.5959) construction
  arc A27 (-58.6236, 8.3323) -> (-59.6248, 4.5959) centre (-35, 0) ccw construction
  line L92 (-58.6236, 8.3323) -> (-60.974, 9.1877) construction
  line L93 (-60.974, 9.1877) -> (-60.803, 9.6576) construction
  line L94 (-60.803, 9.6576) -> (-58.4526, 8.8021) construction
  arc A28 (-56.8179, 12.3079) -> (-58.4526, 8.8021) centre (-35, 0) ccw construction
  line L95 (-56.8179, 12.3079) -> (-58.984, 13.5585) construction
  line L96 (-58.984, 13.5585) -> (-58.734, 13.9915) construction
  line L97 (-58.734, 13.9915) -> (-56.5679, 12.7409) construction
  arc A29 (-54.3492, 15.9095) -> (-56.5679, 12.7409) centre (-35, 0) ccw construction
  line L98 (-54.3492, 15.9095) -> (-56.2652, 17.5173) construction
  line L99 (-56.2652, 17.5173) -> (-55.9438, 17.9003) construction
  line L100 (-55.9438, 17.9003) -> (-54.0278, 16.2925) construction
  arc A30 (-51.2925, 19.0278) -> (-54.0278, 16.2925) centre (-35, 0) ccw construction
  line L101 (-51.2925, 19.0278) -> (-52.9003, 20.9438) construction
  line L102 (-52.9003, 20.9438) -> (-52.5173, 21.2652) construction
  line L103 (-52.5173, 21.2652) -> (-50.9095, 19.3492) construction
  arc A31 (-47.7409, 21.5679) -> (-50.9095, 19.3492) centre (-35, 0) ccw construction
  line L104 (-47.7409, 21.5679) -> (-48.9915, 23.734) construction
  line L105 (-48.9915, 23.734) -> (-48.5585, 23.984) construction
  line L106 (-48.5585, 23.984) -> (-47.3079, 21.8179) construction
  arc A32 (-43.8021, 23.4526) -> (-47.3079, 21.8179) centre (-35, 0) ccw construction
  line L107 (-43.8021, 23.4526) -> (-44.6576, 25.803) construction
  line L108 (-44.6576, 25.803) -> (-44.1877, 25.974) construction
  line L109 (-44.1877, 25.974) -> (-43.3323, 23.6236) construction
  arc A33 (-39.5959, 24.6248) -> (-43.3323, 23.6236) centre (-35, 0) ccw construction
  line L110 (-39.5959, 24.6248) -> (-40.0302, 27.088) construction
  line L111 (-40.0302, 27.088) -> (-39.5378, 27.1749) construction
  line L112 (-39.5378, 27.1749) -> (-39.1035, 24.7116) construction
  arc A34 (-35.25, 25.0488) -> (-39.1035, 24.7116) centre (-35, 0) ccw construction
  line L113 (-35.25, 25.0488) -> (-35.25, 30.8773) construction
  line L114 (-35.25, 30.8773) -> (-34.75, 30.8773) construction
  line L115 (-34.75, 30.8773) -> (-34.75, 25.0488) construction
  arc A35 (-30.8965, 24.7116) -> (-34.75, 25.0488) centre (-35, 0) ccw construction
  line L116 (-30.8965, 24.7116) -> (-30.4622, 27.1749) construction
  line L117 (-30.4622, 27.1749) -> (-29.9698, 27.088) construction
  arc A36 (-70, 0) -> (0, 0) centre (-35, 0) ccw construction
  line L118 (0, 44.9917) -> (0, 0) construction
  line L119 (-70, 44.9917) -> (0, 44.9917) construction
  line L120 (-70, 0) -> (-70, 44.9917) construction
  circle A37 centre (-35, 0) radius 30 construction
  circle A38 centre (-65, 0) radius 1.325
  circle A39 centre (-59.2705, -17.6336) radius 1.325
  circle A40 centre (-44.2705, -28.5317) radius 1.325
  circle A41 centre (-25.7295, -28.5317) radius 1.325
  circle A42 centre (-10.7295, -17.6336) radius 1.325
  circle A43 centre (-5, 0) radius 1.325
  dimension "d55" = 2.65
  dimension "d58" = 180
  constraints: 6 centre point, 1 coincident, 1 horizontal alignment, 22 other
  measures "d55" diameter of A38
extrude "Extrusion12" cut sketch "Skizze13" against normal through all
